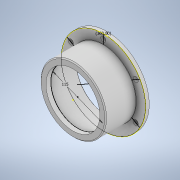
# Autodesk Inventor part: Деталь2
Saved by Autodesk Inventor 2021.2 (Build 252289000, 289)
## iProperties
Created: 2024-04-10
Part Number: Деталь2
Material: Типовые
Document SubType Name: Modeling
Designer: student
Density: 1 g/cm^3
Appearance: По умолчанию
Author: student
Autodesk Inventor part; units mm, degrees
ref_plane "YZ Plane" through (0, 0, 0) normal (1, 0, 0) x (0, 1, 0)
ref_plane "XZ Plane" through (0, 0, 0) normal (0, 1, 0) x (-1, 0, 0)
ref_plane "XY Plane" through (0, 0, 0) normal (0, 0, 1) x (1, 0, 0)
sketch "Эскиз1" plane through (0, 0, 0) normal (0, 0, 1) x (1, 0, 0)
  circle A0 centre (0, 0) radius 90
  dimension "d0" = 180
  constraints: 1 centre point, 1 coincident
  measures "d0" diameter of A0
extrude "Выдавливание1" add sketch "Эскиз1" along normal blind 8
sketch "Эскиз2" plane through (0, 0, 8) normal (0, 0, 1) x (1, 0, 0)
  point P0 (0, 0)
sketch "Эскиз3" plane through (0, 0, 8) normal (0, 0, 1) x (1, 0, 0)
  circle A0 centre (0, 0) radius 70
  dimension "d4" = 140
  constraints: 1 centre point, 1 coincident
  measures "d4" diameter of A0
extrude "Выдавливание2" add sketch "Эскиз3" along normal blind 65
sketch "Эскиз4" plane through (0, 0, 0) normal (0, 0, -1) x (-1, 0, 0)
  circle A0 centre (0, 0) radius 65
  dimension "d7" = 130
  constraints: 1 centre point, 1 coincident
  measures "d7" diameter of A0
extrude "Выдавливание3" cut sketch "Эскиз4" against normal blind 63
chamfer "Фаска1" distance 1 angle 45 1 edges at (65, 0, 0)
chamfer "Фаска2" distance 2 angle 45 1 edges at (-70, 0, 73)
sketch "Эскиз5" plane through (0, 0, 8) normal (0, 0, 1) x (1, 0, 0)
  line L0 (0, 0) -> (0, 90)
  circle A0 centre (0, 0) radius 90 projected
  line L1 (0, 0) -> (-77.9423, 45)
  line L2 (0, 0) -> (-77.9423, -45)
  line L3 (0, 0) -> (0, -90)
  line L4 (0, 0) -> (77.9423, -45)
  line L5 (0, 0) -> (77.9423, 45)
  dimension "d18" = 360
  constraints: 12 end point, 2 coincident, 1 vertical, 1 vertical alignment, 18 other
sketch "Эскиз6" plane through (0, 0, 8) normal (0, 0, 1) x (1, 0, 0)
  point P0 (0, 0)
sketch "Эскиз7" plane through (0, 0, 8) normal (0, 0, 1) x (1, 0, 0)
  point P0 (0, 0)
sketch "Эскиз8" plane through (0, 0, 8) normal (0, 0, 1) x (1, 0, 0)
  point P0 (0, 0)
sketch "Эскиз9" plane through (0, 0, 73) normal (0, 0, 1) x (1, 0, 0)
  point P0 (0, 0)
sketch "Эскиз10" plane through (0, 0, 73) normal (0, 0, 1) x (1, 0, 0)
  circle A0 centre (0, 0) radius 57.5
  dimension "d20" = 115
  constraints: 1 centre point, 1 coincident
  measures "d20" diameter of A0
sketch "Эскиз11" plane through (0, 0, 63) normal (0, 0, -1) x (-1, 0, 0)
  circle A0 centre (0, 0) radius 57.5
  dimension "d21" = 115
  constraints: 1 centre point, 1 coincident
  measures "d21" diameter of A0
hole "Отверстие1" at (0, 0, 73) direction (0, 0, -1) diameter 115 end through all
sketch "Эскиз12" plane through (0, 0, 8) normal (0, 0, 1) x (1, 0, 0)
  circle A0 centre (0, 0) radius 80
  circle A1 centre (0, 0) radius 70 projected
  point P0 (0, 80)
  point P1 (-69.282, 40)
  point P2 (-69.282, -40)
  point P3 (0, -80)
  point P4 (69.282, -40)
  point P5 (69.282, 40)
  dimension "d29" = 160
  dimension "d32" = 360
  constraints: 2 coincident, 1 vertical alignment, 9 other
hole "Отверстие2" at (0, 80, 8) at (69.282, 40, 8) at (69.282, -40, 8) at (0, -80, 8) at (-69.282, -40, 8) at (-69.282, 40, 8) direction (0, 0, -1) diameter 11 end through all
fillet "Сопряжение1" radius 0.6 1 edges at (-70, 0, 8)
